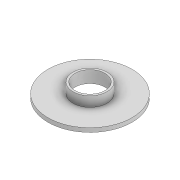
# Autodesk Inventor part: Seal_M
Saved by Autodesk Inventor 2020 (Build 240168000, 168)
## iProperties
Created: 2020-04-30
Part Number: Seal_M
Material: Generic
Document SubType Name: Modeling
Designer: Theo Cominotto
Density: 1 g/cm^3
Appearance: Default
d0: 1,500 mm
d1: 1,500 mm
d2: 20,000 mm
d3: 1,500 mm
d4: 14,500 mm
d6: 8,500 mm
d7: 1,000 mm
d8: 6,000 mm
d9: 1,000 mm
d10: 1,000 mm
d11: 1,000 mm
d13: 0,500 mm
Author: Theo Cominotto
Autodesk Inventor part; units mm, degrees
ref_plane "YZ Plane" through (0, 0, 0) normal (1, 0, 0) x (0, 1, 0)
ref_plane "XZ Plane" through (0, 0, 0) normal (0, 1, 0) x (-1, 0, 0)
ref_plane "XY Plane" through (0, 0, 0) normal (0, 0, 1) x (1, 0, 0)
sketch "Sketch1" plane through (0, 0, 0) normal (0, 0, 1) x (1, 0, 0)
  line L0 (0, 0) -> (1.5, 0) construction
  line L1 (1.5, 0) -> (1.5, 1.5) construction
  line L2 (1.5, 1.5) -> (0, 1.5) construction
  line L3 (0, 0) -> (20, 0) construction
  line L4 (20, 0) -> (20, 1.5)
  line L5 (0, 0) -> (14.5, 0) construction
  line L6 (20, 1.5) -> (7.5, 1.5)
  line L7 (0, 1.5) -> (8.5, 1.5) construction
  line L8 (0, -1.5) -> (0, 9) construction
  line L9 (7.5, 1.5) -> (7.5, 7.5)
  line L10 (7.5, 7.5) -> (8.5, 7.5)
  line L11 (8.5, 7.5) -> (8.5, 2.5)
  line L12 (8.5, 2.5) -> (21, 2.5)
  line L13 (21, 2.5) -> (21, 0)
  line L14 (21, 0) -> (20, 0)
  line L15 (20, 0) -> (21, 0)
  line L16 (21, 0) -> (21, 0.5)
  line L17 (21, 0.5) -> (20, 0.5)
  line L18 (20, 0.5) -> (20, 0)
  dimension "d0" = 1.5
  dimension "d1" = 1.5
  dimension "d2" = 20
  dimension "d3" = 1.5
  dimension "d4" = 14.5
  dimension "d6" = 8.5
  dimension "d7" = 1
  dimension "d8" = 6
  dimension "d9" = 1
  dimension "d10" = 1
  dimension "d11" = 1
  dimension "d13" = 0.5
  constraints: 36 end point, 8 perpendicular, 5 horizontal, 3 point on line, 2 parallel, 2 vertical, 1 collinear
  measures "d0" distance of L0.start L0.end
  measures "d1" distance of L0.end L1.end
  measures "d2" distance of L0.start L3.end
  measures "d3" distance of L3.end L4.end
  measures "d4" distance of L0.start L5.end
  measures "d6" distance of L7.start L7.end
  measures "d7" distance of L7.end L6.end
  measures "d8" distance of L6.end L9.end
  measures "d9" distance of L9.end L10.end
  measures "d10" distance between parallel lines of L6 L12
  measures "d11" distance between parallel lines of L4 L13
  measures "d13" distance between parallel lines of L14 L17
revolve "Revolution2" add sketch "Sketch1" angle 360 about axis through (0, -10, 0) along (0, 1, 0) contours L4 L6 L9 L10 L11 L12 L13 L17
body "Solid2"
